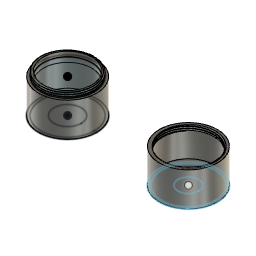
_AutoBulbCase.8b675a72-df1e-4321-84a9-f24b0cf54006 (Autodesk Fusion 360 design; units mm, degrees)
Autodesk Fusion 360 part; units mm, degrees
sketch "Sketch1" plane through (0, 0, 0) normal (0, 0, 1) x (1, 0, 0)
  circle A0 centre (0, 0) radius 30
  circle A1 centre (125, 0) radius 30
  circle A2 centre (0, 0) radius 27.5
  circle A3 centre (125, 0) radius 27.5
  circle A4 centre (0, 0) radius 14
  circle A5 centre (125, 0) radius 10.5
  dimension "d17" = 60
  dimension "d18" = 60
  dimension "d19" = 55
  dimension "d20" = 55
  dimension "d21" = 28
  dimension "d22" = 21
  constraint coincident A0.centre A2.centre
  constraint concentric A0 A2
  constraint concentric A1 A3
  constraint concentric A3 A5
  measures "d17" diameter of A0
  measures "d18" diameter of A1
  measures "d19" diameter of A2
  measures "d20" diameter of A3
  measures "d21" diameter of A4
  measures "d22" diameter of A5
extrude "Extrude5" add sketch "Sketch1" along normal blind 5 contours A2 | A3 makes body 1 at (22.8455, -2.0618, 0) makes body 2 at (146.6919, -1.8879, 0)
extrude "Extrude6" add sketch "Sketch1" along normal blind 35 contours A0 | A1 bodies 1 2
ref_plane "WorkPlane1" through (0, 0, 35) normal (0, 0, 1) x (1, 0, 0)
sketch "Sketch2" plane through (0, 0, 35) normal (0, 0, 1) x (1, 0, 0)
  circle A0 centre (0, 0) radius 25
  circle A1 centre (0, 0) radius 27.5
  dimension "d28" = 50
  dimension "d29" = 55
  constraint coincident A0.centre A1.centre
  measures "d28" diameter of A0
  measures "d29" diameter of A1
extrude "Extrude7" add sketch "Sketch2" against normal blind 5 bodies 1
extrude "Extrude8" add sketch "Sketch2" along normal blind 5 bodies 1
thread "Thread7" "ISO Metric profile 55.0 M55x2 6H" major diameter 55.2623 minor diameter 53.0224 pitch 2 angle 60 modelled right hand crest width 0.5401 on face at (152.3633, -2.7381, 25) from (125, 0, 30) to (125, 0, 35) crest through (151.5112, 0, 5.5) on bodies 2
thread "Thread8" "ISO Metric profile 55.0 M55x2 6g" major diameter 54.822 minor diameter 52.5239 pitch 2 angle 60 modelled right hand crest width 0.2789 on face at (27.4658, -1.3708, 38.3333) crest through (27.411, 0, 34.5) on bodies 1
thread "Thread9" "ISO Metric profile 28.0 M28x1.5 6H" major diameter 28.2083 minor diameter 26.5262 pitch 1.5 angle 60 modelled right hand crest width 0.4039 on face at (13.9826, -0.6978, 3.3333) crest through (13.2631, 0, 0.375) on bodies 1
thread "Thread10" "ISO Metric profile 20.0 M20x1.5 6H" major diameter 20.203 minor diameter 18.526 pitch 1.5 angle 60 modelled right hand crest width 0.4065 on face at (135.4869, 0.5234, 1.6667) crest through (134.263, 0, 0.375) on bodies 2
